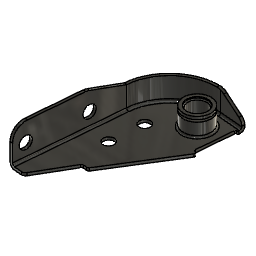
bracket for clutch v1 (Autodesk Fusion 360 design; units mm, degrees)
Autodesk Fusion 360 part; units mm, degrees
note: some values were not read from the file. Chosen so that the rebuilt part matches the saved one: which bodies a step acts on; a direction. Set by a fixed rule: which sketch regions a step uses; which face or edge a step refers to.
sketch "Sketch1" plane through (0, 0, 0) normal (0, 0, 1) x (1, 0, 0)
  line L0 (0, 0) -> (140, 0)
  line L1 (140, 0) -> (140, -66)
  line L2 (140, -66) -> (134, -66)
  line L3 (134, -66) -> (134, -64)
  line L4 (134, -64) -> (99, -64)
  line L5 (0, 0) -> (0, -13.5)
  line L6 (0, 0) -> (35, 0)
  line L7 (0, -13.5) -> (35, -30)
  line L8 (35, -30) -> (35, -35.5)
  line L9 (99, -64) -> (99, -68)
  line L10 (99, -68) -> (35, -35.5)
  dimension "d1" = 140
  dimension "d4" = 35
  dimension "d5" = 13.5
  dimension "d6" = 35
  dimension "d7" = 30
  dimension "d8" = 5.5
  constraint coincident L0.start L5.start
  constraint horizontal L0
  constraint perpendicular L0 L1
  constraint perpendicular L1 L2
  constraint perpendicular L2 L3
  constraint perpendicular L3 L4
  constraint perpendicular L0 L5
  constraint parallel L0 L6
  constraint perpendicular L6 L8
  constraint perpendicular L4 L9
  measures "d1" distance of L0.start L0.end
  measures "d4" distance of L3.end L4.end
  measures "d5" distance of L0.start L5.end
  measures "d6" distance of L0.start L6.end
  measures "d7" distance of L6.end L7.end
  measures "d8" distance of L7.end L8.end
extrude "Extrude1" add sketch "Sketch1" along normal blind 2.5 makes body 1
fillet "Fillet1" radius 1.5 2 edges at (99, -64, 1.25) (99, -68, 1.25) on bodies 1
fillet "Fillet2" radius 1 2 edges at (134, -64, 1.25) (134, -66, 1.25) on bodies 1
fillet "Fillet3" radius 2 2 edges at (35, -30, 1.25) (35, -35.5, 1.25) on bodies 1
fillet "Fillet4" radius 3.5 1 edges at (0, -13.5, 1.25) on bodies 1
fillet "Fillet5" radius 45 1 edges at (140, 0, 1.25) on bodies 1
sketch "Sketch2" plane through (0, 0, 2.5) normal (0, 0, 1) x (-1, 0, 0)
  arc A0 (-140, 45) -> (-95, 0) centre (-95, 45) ccw
  line L0 (-95, 0) -> (0, 0)
  line L1 (0, 0) -> (0, 11.2806)
  arc A1 (0, 11.2806) -> (-2.0075, 14.4464) centre (-3.5, 11.2806) ccw
  line L2 (-2.0075, 14.4464) -> (-33.8528, 29.4592)
  arc A2 (-35, 31.2682) -> (-33.8528, 29.4592) centre (-33, 31.2682) ccw
  line L3 (-35, 31.2682) -> (-35, 34.2725)
  arc A3 (-35, 34.2725) -> (-36.0944, 36.0558) centre (-37, 34.2725) ccw
  line L4 (-36.0944, 36.0558) -> (-96.8208, 66.8934)
  arc A4 (-96.8208, 66.8934) -> (-99, 65.556) centre (-97.5, 65.556) ccw
  line L5 (-99, 65.556) -> (-99, 65.5)
  arc A5 (-100.5, 64) -> (-99, 65.5) centre (-100.5, 65.5) ccw
  line L6 (-100.5, 64) -> (-133, 64)
  arc A6 (-134, 65) -> (-133, 64) centre (-133, 65) ccw
  arc A7 (-134, 65) -> (-135, 66) centre (-135, 65) ccw
  line L7 (-135, 66) -> (-140, 66)
  line L8 (-140, 66) -> (-140, 45)
  line L9 (-137.5, 66) -> (-137.5, 45)
  arc A8 (-137.5, 45) -> (-95, 2.5) centre (-95, 45) ccw
  line L10 (-95, 2.5) -> (0, 2.5)
  line L11 (-137.5, 66) -> (-140, 66)
  line L12 (0, 0) -> (0, 2.5)
  dimension "d22" = -2.5
  constraint coincident L7.end L8.start
  constraint perpendicular L8 L11
  constraint coincident L0.end L1.start
  constraint perpendicular L10 L12
extrude "Extrude2" add sketch "Sketch2" along normal blind 30 contours A0 L0 L1 L7 L8 L9 A8 L10 L11 L12 bodies 1
fillet "Fillet6" radius 12.5 1 edges at (0, -1.25, 32.5) on bodies 1
sketch "Sketch3" plane through (0, -2.5, 0) normal (0, -1, 0) x (1, 0, 0)
  arc A0 (12.5, 32.5) -> (0, 20) centre (12.5, 20) ccw
  line L0 (0, 20) -> (0, 2.5)
  line L1 (0, 2.5) -> (95, 2.5)
  line L2 (95, 2.5) -> (95, 32.5)
  line L3 (95, 32.5) -> (12.5, 32.5)
  line L4 (95, 32.5) -> (95, 22.5)
  line L5 (12.5, 32.5) -> (62.5, 32.5)
  line L6 (62.5, 32.5) -> (95, 22.5)
  line L7 (95, 32.5) -> (154.12, 32.5)
  line L8 (154.12, 32.5) -> (154.12, 22.5)
  line L9 (154.12, 22.5) -> (95, 22.5)
  line L10 (95, 22.5) -> (95, 32.5)
  dimension "d27" = 10
  dimension "d28" = 50
  constraint coincident L2.end L3.start
  constraint perpendicular L3 L4
  constraint coincident A0.start L3.end
  constraint parallel L3 L5
  constraint horizontal L7
  constraint vertical L8
  constraint horizontal L9
  constraint vertical L10
  measures "d27" distance of L2.end L4.end
  measures "d28" distance of A0.start L5.end
extrude "Extrude3" cut sketch "Sketch3" along normal blind 105 contours L2 L3 L4 L6 L10 | L2 L4 L7 L8 L9 L10 bodies 1
extrude "Extrude4" cut sketch "Sketch3" against normal blind 50 contours L2 L3 L4 L6 L10 | L2 L4 L7 L8 L9 L10 bodies 1
sketch "Sketch4" plane through (137.5, 0, 0) normal (-1, 0, 0) x (0, -1, 0)
  line L0 (66, 22.5) -> (45, 22.5)
  line L1 (45, 22.5) -> (45, 2.5)
  line L2 (45, 2.5) -> (66, 2.5)
  line L3 (66, 2.5) -> (66, 22.5)
  line L4 (66, 2.5) -> (66, 8.5)
  line L5 (45, 22.5, -2.5) -> (66, 22.5, -2.5)
  line L6 (66, 8.5) -> (45, 22.5)
  line L7 (66, 22.5) -> (66, 8.5)
  point P0 (45, 22.5)
  point P1 (66, 22.5)
  dimension "d33" = 6
  constraint coincident L2.end L3.start
  constraint perpendicular L2 L4
  constraint coincident P0 L0.end
  constraint coincident P1 L0.start
  constraint coincident L0.start L3.end
  measures "d33" distance of L2.end L4.end
extrude "Extrude5" cut sketch "Sketch4" against normal blind 35 contours L0 L3 L6 L7 bodies 1
fillet "Fillet7" radius 11 1 edges at (62.5, -1.25, 32.5) on bodies 1
fillet "Fillet8" radius 12 1 edges at (138.75, -45, 22.5) on bodies 1
fillet "Fillet9" radius 6.5 1 edges at (138.75, -66, 8.5) on bodies 1
fillet "Fillet10" radius 4 3 edges at (140, -55.5, 0) (126.8198, -13.1802, 0) (47.5, 0, 0) on bodies 1
fillet "Fillet11" radius 2 3 edges at (137.5, -55.5, 2.5) (125.052, -14.948, 2.5) (47.5, -2.5, 2.5) on bodies 1
sketch "Sketch5" plane through (0, -2.5, 0) normal (0, -1, 0) x (1, 0, 0)
  line L0 (0, 4.5) -> (95, 4.5)
  line L1 (95, 4.5) -> (95, 22.5)
  line L2 (95, 22.5) -> (64.0809, 32.0136)
  arc A0 (64.0809, 32.0136) -> (60.846, 32.5) centre (60.846, 21.5) ccw
  line L3 (60.846, 32.5) -> (12.5, 32.5)
  arc A1 (12.5, 32.5) -> (0, 20) centre (12.5, 20) ccw
  line L4 (0, 20) -> (0, 4.5)
  line L5 (12.5, 32.5) -> (12.5, 15.5)
  line L6 (12.5, 15.5) -> (50, 15.5)
  line L7 (50, 15.5) -> (2, 15.5)
  line L8 (50, 15.5) -> (82.6187, 15.5)
  line L9 (0, 15.5) -> (11, 15.5)
  circle A2 centre (11, 15.5) radius 5.5
  line L10 (64.0809, 32.0136) -> (64.0809, 15.5)
  circle A3 centre (64.0809, 15.5) radius 5.5
  dimension "d46" = 17
  dimension "d47" = 11
  dimension "d48" = 11
  constraint coincident L3.end A1.start
  constraint perpendicular L0 L5
  constraint perpendicular L5 L6
  constraint perpendicular L5 L7
  constraint parallel L7 L8
  constraint coincident L4 L9.start
  constraint coincident L7 L9.end
  constraint coincident L9.end A2.centre
  constraint coincident L2.end A0.start
  constraint coincident L8 L10.end
  constraint perpendicular L8 L10
  constraint coincident L10.end A3.centre
  measures "d46" distance of L3.end L5.end
  measures "d47" diameter of A2
  measures "d48" diameter of A3
extrude "Extrude6" cut sketch "Sketch5" against normal blind 21 contours L5 L7 L9 A2 | L6 L7 L9 A2 | L8 L10 A3 | L8 L10 A3 | L5 L6 L7 A2 | L8 A3 bodies 1
sketch "Sketch6" plane through (0, 0, 2.5) normal (0, 0, 1) x (-1, 0, 0)
  circle A0 through (-69.5809, 2.5, 13) (-61.3309, 2.5, 17.7631) (-61.3309, 2.5, 8.2369)
  line L0 (-64.0809, 2.5, 13) -> (-64.0809, 21.5, 13)
  circle A1 through (-59.0809, 21.5, 13) (-66.5809, 25.8301, 13) (-66.5809, 17.1699, 13)
  dimension "d51" = 19
  dimension "d52" = 10
sketch "Sketch7" plane through (0, 0, 15.5) normal (0, 0, 1) x (-1, 0, 0)
  line L0 (-64.0809, 21.5) -> (-94.0809, 21.5)
  circle A0 centre (-94.0809, 21.5) radius 5
  point P0 (-64.0809, 21.5)
  dimension "d53" = 30
  dimension "d54" = 10
  constraint coincident P0 L0.start
  constraint horizontal L0
  constraint coincident L0.end A0.centre
  measures "d53" distance of P0 L0.end
  measures "d54" diameter of A0
sketch "Sketch6 (curves 13 mm off its plane)" plane through (0, 0, 15.5) normal (0, 0, 1) x (-1, 0, 0)
  line L0 (-64.0809, 2.5) -> (-64.0809, 21.5)
  circle A0 centre (-64.0809, 21.5) radius 5
extrude "Extrude7" cut sketch "Sketch7" sketch "Sketch6 (curves 13 mm off its plane)" against normal blind 25 of sketch 2 bodies 1
sketch "Sketch8" plane through (0, 0, 2.5) normal (0, 0, 1) x (-1, 0, 0)
  line L0 (-100.5, 64) -> (-133, 64)
  line L1 (-116.75, 64) -> (-116.75, 45)
  line L2 (-140, 45) -> (-118, 45)
  circle A0 centre (-118, 45) radius 12.5
  point P0 (-140, 45)
  dimension "d57" = 19
  dimension "d58" = 22
  dimension "d59" = 25
  constraint midpoint L0 L1.start
  constraint perpendicular L0 L1
  constraint coincident P0 L2.start
  constraint perpendicular L1 L2
  constraint coincident L2.end A0.centre
  measures "d57" distance of L1.start L1.end
  measures "d58" distance of P0 L2.end
  measures "d59" diameter of A0
extrude "Extrude8" add sketch "Sketch8" along normal blind 16.5 thin wall 4 inside bodies 1
sketch "Sketch9" plane through (0, 0, 19) normal (0, 0, 1) x (-1, 0, 0)
  circle A0 centre (-118, 45) radius 8.5
  circle A1 centre (-118, 45) radius 12.5
  circle A2 centre (-118, 45) radius 9.5
  dimension "d63" = 1
extrude "Extrude9" cut sketch "Sketch9" against normal blind 4 contours A2 bodies 1
sketch "Sketch10" plane through (0, 0, 19) normal (0, 0, 1) x (-1, 0, 0)
  circle A0 centre (-118, 45) radius 9.5
  circle A1 centre (-118, 45) radius 12.5
  line L0 (-119.0335, 54.4436, 0) -> (-119.0335, 54.4436, -2.5)
  line L1 (-119.0335, 54.4436, -2.5) -> (-104.0335, 54.4436, -2.5)
  line L2 (-104.0335, 54.4436, -2.5) -> (-104.0335, 54.4436, -4.5)
  line L3 (-104.0335, 54.4436, -4.5) -> (-119.0335, 54.4436, -4.5)
  line L4 (-119.0335, 54.4436, -4.5) -> (-119.0335, 54.4436, -2.5)
  line L5 (-119.0335, 54.4436, -2.5) -> (-134.0335, 54.4436, -2.5)
  line L6 (-134.0335, 54.4436, -2.5) -> (-134.0335, 54.4436, -4.5)
  line L7 (-134.0335, 54.4436, -4.5) -> (-119.0335, 54.4436, -4.5)
  line L8 (-119.0335, 54.4436, -4.5) -> (-119.0335, 54.4436, -2.5)
  dimension "d66" = 2.5
  dimension "d67" = 15
  dimension "d68" = 2
  dimension "d69" = 15
sketch "Sketch10 (curves on the plane with normal 0, -1, 0 at 54.4436 mm)" plane through (0, -54.4436, 19) normal (0, -1, 0) x (1, 0, 0)
  line L0 (119.0335, 0) -> (119.0335, -2.5)
  line L1 (119.0335, -2.5) -> (104.0335, -2.5)
  line L2 (104.0335, -2.5) -> (104.0335, -4.5)
  line L3 (104.0335, -4.5) -> (119.0335, -4.5)
  line L4 (119.0335, -4.5) -> (119.0335, -2.5)
  line L5 (119.0335, -2.5) -> (134.0335, -2.5)
  line L6 (134.0335, -2.5) -> (134.0335, -4.5)
  line L7 (134.0335, -4.5) -> (119.0335, -4.5)
  line L8 (119.0335, -4.5) -> (119.0335, -2.5)
extrude "Extrude10" cut sketch "Sketch10 (curves on the plane with normal 0, -1, 0 at 54.4436 mm)" against normal blind 5 and the other way blind 25 bodies 1
extrude "Extrude12" cut 1 faces at (107.4121, -49.4436, 15.3333) along direction (0, 1, 0) blind 25 on bodies 1 bodies 1
sketch "Sketch11" plane through (0, 0, 19) normal (0, 0, 1) x (-1, 0, 0)
  line L0 (-104.0335, 54.4436, -2.5) -> (-104.0335, 26.2845, -2.5)
  line L1 (-104.0335, 26.2845, -2.5) -> (-104.0335, 26.2845, -4.5)
  line L2 (-104.0335, 26.2845, -4.5) -> (-104.0335, 54.4436, -4.5)
  line L3 (-104.0335, 54.4436, -4.5) -> (-104.0335, 54.4436, -2.5)
  point P0 (-104.0335, 54.4436)
sketch "Sketch11 (curves on the plane with normal -1, 0, 0 at -104.0335 mm)" plane through (104.0335, 0, 19) normal (-1, 0, 0) x (0, -1, 0)
  line L0 (54.4436, -2.5) -> (26.2845, -2.5)
  line L1 (26.2845, -2.5) -> (26.2845, -4.5)
  line L2 (26.2845, -4.5) -> (54.4436, -4.5)
  line L3 (54.4436, -4.5) -> (54.4436, -2.5)
extrude "Extrude13" cut sketch "Sketch11 (curves on the plane with normal -1, 0, 0 at -104.0335 mm)" against normal blind 28 bodies 1 makes body 2 at (111.0937, -42.8581, 0)
extrude "Extrude14" add sketch "Sketch9" along normal blind -2.5 and the other way blind 7 contours A2 bodies 2 1
extrude "Extrude15" add 1 faces at (108.9003, -44.1057, 16.5) along direction (0, 0, 1) blind 0.5 on bodies 2 bodies 2
fillet "Fillet12" radius 1 1 edges at (126.8571, -48.4353, 17) on bodies 2
move_body "Move1" bodies 2 to x (0.087156, 0.996195, 0) y (-0.996195, 0.087156, 0) z (0, 0, 1) at (-0.3669, -68.1447, 0)
fillet "Fillet13" radius 1.5 1 edges at (60.265, 56.7001, 2.5) on bodies 2
